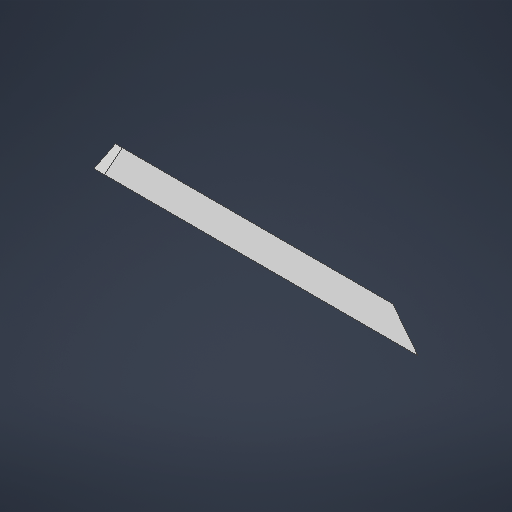
# Autodesk Inventor part: SS_2x4x51.684
Saved by Autodesk Inventor 2026 (Build 300175000, 175)
## iProperties
Created: 2025-09-04
Part Number: SS_2x4x51.684
Material: Generic
Document SubType Name: Modeling
Designer: trott
Density: 1 g/cm^3
Appearance: Default
Author: trott
Autodesk Inventor part; units mm, degrees
ref_plane "YZ Plane" through (0, 0, 0) normal (1, 0, 0) x (0, 1, 0)
ref_plane "XZ Plane" through (0, 0, 0) normal (0, 1, 0) x (-1, 0, 0)
ref_plane "XY Plane" through (0, 0, 0) normal (0, 0, 1) x (1, 0, 0)
sketch "Sketch1" plane through (0, 0, 0) normal (0, 0, 1) x (1, 0, 0)
  line L0 (0, 0) -> (304.8, 0)
  line L1 (0, 0) -> (0, 914.4)
  line L2 (0, 914.4) -> (304.8, 0)
  line L3 (304.8, 0) -> (340.9448, 12.0483)
  line L4 (0, 914.4) -> (36.1448, 926.4483)
  line L5 (340.9448, 12.0483) -> (36.1448, 926.4483)
  line L6 (0, 914.4) -> (0, 1066.8)
  line L7 (0, 1066.8) -> (457.2, 1066.8)
  line L8 (457.2, 1066.8) -> (457.2, 0)
  line L9 (457.2, 0) -> (304.8, 0)
  line L10 (36.1448, 926.4483) -> (0, 1034.8828)
  line L11 (340.9448, 12.0483) -> (344.9609, 0)
  line L12 (0, 1034.8828) -> (-36.1448, 1022.8345)
  line L13 (-36.1448, 1022.8345) -> (0, 914.4)
  line L14 (344.9609, 0) -> (308.8161, -12.0483)
  line L15 (304.8, 0) -> (308.8161, -12.0483)
  dimension "d34" = 304.8
  dimension "d35" = 914.4
  dimension "d36" = 38.1
  dimension "d37" = 38.1
  dimension "d38" = 152.4
  dimension "d39" = 457.2
  dimension "d40" = 1066.8
  dimension "d45" = 38.1
  dimension "d46" = 38.1
  constraints: 32 end point, 5 perpendicular, 3 vertical, 2 collinear, 2 point on line, 1 horizontal
  measures "d34" distance of L0.start L0.end
  measures "d35" distance of L0.start L1.end
  measures "d36" distance of L0.end L3.end
  measures "d37" distance of L1.end L4.end
  measures "d38" distance of L1.end L6.end
  measures "d39" distance of L6.end L7.end
  measures "d40" distance of L7.end L8.end
  measures "d45" distance of L10.end L12.end
  measures "d46" distance of L11.end L14.end
sketch "Sketch2" plane through (0, 0, 0) normal (1, 0, 0) x (0, 1, 0)
  line L0 (0, 0) -> (0, 914.4)
  line L1 (0, 914.4) -> (914.4, 914.4)
  line L2 (914.4, 914.4) -> (914.4, 0)
  line L3 (914.4, 914.4) -> (0, 0)
  line L4 (914.4, 914.4) -> (977.2618, 851.5382)
  line L5 (0, 0) -> (62.8618, -62.8618)
  line L6 (977.2618, 851.5382) -> (914.4, 788.6764)
  line L7 (914.4, 0) -> (366.5441, 0)
  line L8 (914.4, 0) -> (1219.2, 0)
  line L9 (0, 0) -> (0, -609.6)
  line L10 (914.4, 0) -> (914.4, 304.8)
  line L11 (914.4, 304.8) -> (1219.2, 304.8)
  line L12 (1219.2, 304.8) -> (1219.2, 0)
  line L13 (1219.2, 304.8) -> (914.4, 914.4)
  line L14 (1219.2, 304.8) -> (914.4, 228.6)
  line L15 (167.6314, 41.9079) -> (0, 0)
  line L16 (167.6314, 41.9079) -> (125.7236, 0)
  line L17 (1219.2, 304.8) -> (1240.7614, 218.5543)
  line L18 (0, 0) -> (21.5614, -86.2457)
  line L19 (21.5614, -86.2457) -> (366.5441, 0)
  line L20 (366.5441, 0) -> (914.4, 136.964)
  line L21 (914.4, 136.964) -> (1240.7614, 218.5543)
  line L22 (914.4, 228.6) -> (167.6314, 41.9079)
  line L23 (366.5441, 0) -> (125.7236, 0)
  line L24 (125.7236, 0) -> (62.8618, -62.8618)
  line L25 (125.7236, 0) -> (0, 0)
  line L26 (914.4, 788.6764) -> (167.6314, 41.9079)
  line L27 (1219.2, 304.8) -> (1219.2, 914.4)
  line L28 (1219.2, 914.4) -> (914.4, 914.4)
  line L29 (21.5614, -86.2457) -> (0, -91.636)
  line L30 (0, -609.6) -> (0, -914.4)
  line L31 (0, -914.4) -> (1219.2, -914.4)
  line L32 (1219.2, -914.4) -> (1219.2, 0)
  line L33 (0, -91.636) -> (-21.5614, -5.3904)
  line L34 (0, 0) -> (-21.5614, -5.3904)
  line L35 (977.2618, 851.5382) -> (977.2618, 304.8)
  line L36 (0, -914.4) -> (-152.4, -914.4)
  line L37 (-152.4, -914.4) -> (-152.4, 914.4)
  line L38 (-152.4, 914.4) -> (0, 914.4)
  point P0 (125.7236, 0)
  point P1 (1219.2, 213.164)
  point P2 (956.3079, 830.5843)
  dimension "d5" = 914.4
  dimension "d6" = 914.4
  dimension "d7" = 914.4
  dimension "d8" = 88.9
  dimension "d9" = 88.9
  dimension "d14" = 304.8
  dimension "d15" = 609.6
  dimension "d16" = 304.8
  dimension "d17" = 304.8
  dimension "d18" = 88.9
  dimension "d24" = 304.8
  dimension "d25" = 1219.2
  dimension "d30" = 88.9
  dimension "d47" = 152.4
  dimension "d48" = 1828.8
  constraints: 78 end point, 15 perpendicular, 7 point on line, 4 vertical, 2 horizontal
  measures "d5" distance of L0.start L0.end
  measures "d6" distance of L0.end L1.end
  measures "d7" distance of L1.end L2.end
  measures "d8" distance of L1.end L4.end
  measures "d9" distance of L0.start L5.end
  measures "d14" distance of L2.end L8.end
  measures "d15" distance of L0.start L9.end
  measures "d16" distance of L2.end L10.end
  measures "d17" distance of L10.end L11.end
  measures "d18" distance of L11.end L17.end
  measures "d24" distance of L9.end L30.end
  measures "d25" distance of L30.end L31.end
  measures "d30" distance of L29.end L33.end
  measures "d47" distance of L30.end L36.end
  measures "d48" distance of L36.end L37.end
extrude "Extrusion7" add sketch "Sketch1" along normal mid plane 1828.8 contours L2 L4 L5 L3 | L3 L11 L9 | L6 L10 L4
extrude "Extrusion8" cut sketch "Sketch2" along normal mid plane 914.4 contours L0 L1 L3 | L25 L24 L5 | L18 L29 L9 | L5 L24 L23 L19 L18 | L15 L16 L25 | L28 L27 L13 L35 L4 | L4 L6 L13 | L29 L19 L7 L8 L32 L31 L30 L9 | L22 L2 L20 L23 L16 | L26 L2 L22 | L6 L13 L35 L11 L2 | L35 L13 L6 | L14 L12 L21 L2 | L2 L11 L14 | L20 L2 L7 | L13 L11 L35 | L21 L12 L8 L2
body "Solid5"
